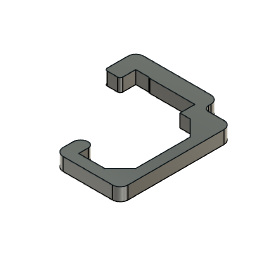
Test frame - motor holders + wheel v4 (Autodesk Fusion 360 archive; units mm, degrees)
design "Single motor Holder"
Autodesk Fusion 360 part; units mm, degrees
note: some values were not read from the file. Chosen so that the rebuilt part matches the saved one: which bodies a step acts on; which face or edge a step refers to. Set by a fixed rule: which sketch regions a step uses.
(part 1 of 2)
sketch "Sketch1" plane through (0, 0, 0) normal (0, 0, 1) x (1, 0, 0)
  line L0 (60.0013, 14) -> (60.0013, 15)
  arc A0 (60.0013, 14) -> (62.0013, 12) centre (62.0013, 14) ccw
  line L1 (51, -27) -> (51, -22.0146)
  line L2 (61, 6) -> (66, 1)
  line L3 (39.0326, 12) -> (39.0326, 11.75)
  line L4 (61, -27) -> (57, -27)
  line L5 (57.0013, 6) -> (61, 6)
  arc A1 (68.0013, -31) -> (71.0013, -28) centre (68.0013, -28) ccw
  line L6 (46, -24.2507) -> (46, -28)
  line L7 (28, 15) -> (28, 6)
  arc A2 (31, 18) -> (28, 15) centre (31, 15) ccw
  line L8 (34, 6) -> (34, 12)
  arc A3 (71.0013, 9) -> (68.0013, 12) centre (68.0013, 9) ccw
  arc A4 (60.0013, 15) -> (57.0013, 18) centre (57.0013, 15) ccw
  arc A5 (46, -28) -> (49, -31) centre (49, -28) ccw
  line L9 (34, 12) -> (39.0326, 12)
  line L10 (68.0013, 12) -> (62.0013, 12)
  line L11 (71.0013, -28) -> (71.0013, 9)
  line L12 (57, 12) -> (57.0013, 12)
  line L13 (39.0326, 11.75) -> (57, 11.75)
  line L14 (49, -31) -> (68.0013, -31)
  line L15 (57.0013, 18) -> (31, 18)
  line L16 (66, 1) -> (66, -22)
  line L17 (28, 6) -> (34, 6)
  line L18 (57, -27) -> (51, -27)
  arc A6 (51, -22.0146) -> (46, -24.2507) centre (49, -24.2507) ccw
  line L19 (66, -22) -> (61, -27)
  line L20 (57.0013, 11.75) -> (57.0013, 6)
  line L21 (57, 11.75) -> (57.0013, 11.75)
  constraint perpendicular L20 L21
extrude "Extrude1" add sketch "Sketch1" along normal blind 5
fillet "Fillet1" radius 1 2 edges at (28, 6, 2.5) (34, 6, 2.5)
fillet "Fillet2" radius 2 1 edges at (51, -22.0146, 2.5)
fillet "Fillet3" radius 1 1 edges at (39.0326, 11.75, 2.5)
sketch "Sketch2" plane through (0, 0, 5) normal (0, 0, 1) x (-1, 0, 0)
  arc A0 (-39.0326, -12) -> (-39.694, -11.75) centre (-39.694, -12.75) ccw
  line L0 (-39.694, -11.75) -> (-57.0013, -11.75)
  line L1 (-57.0013, -11.75) -> (-57.0013, -6)
  line L2 (-57.0013, -6) -> (-61, -6)
  line L3 (-61, -6) -> (-66, -1)
  line L4 (-66, -1) -> (-66, 22)
  line L5 (-66, 22) -> (-61, 27)
  line L6 (-61, 27) -> (-51, 27)
  line L7 (-51, 27) -> (-51, 23.2507)
  arc A1 (-51, 23.2507) -> (-49, 21.2507) centre (-49, 23.2507) ccw
  arc A2 (-49, 21.2507) -> (-46, 24.2507) centre (-49, 24.2507) ccw
  line L8 (-46, 24.2507) -> (-46, 28)
  arc A3 (-46, 28) -> (-49, 31) centre (-49, 28) ccw
  line L9 (-49, 31) -> (-68.0013, 31)
  arc A4 (-68.0013, 31) -> (-71.0013, 28) centre (-68.0013, 28) ccw
  line L10 (-71.0013, 28) -> (-71.0013, -9)
  arc A5 (-71.0013, -9) -> (-68.0013, -12) centre (-68.0013, -9) ccw
  line L11 (-68.0013, -12) -> (-62.0013, -12)
  arc A6 (-60.0013, -14) -> (-62.0013, -12) centre (-62.0013, -14) ccw
  line L12 (-60.0013, -14) -> (-60.0013, -15)
  arc A7 (-60.0013, -15) -> (-57.0013, -18) centre (-57.0013, -15) ccw
  line L13 (-57.0013, -18) -> (-31, -18)
  arc A8 (-31, -18) -> (-28, -15) centre (-31, -15) ccw
  line L14 (-28, -15) -> (-28, -7)
  arc A9 (-28, -7) -> (-29, -6) centre (-29, -7) ccw
  line L15 (-29, -6) -> (-33, -6)
  arc A10 (-33, -6) -> (-34, -7) centre (-33, -7) ccw
  line L16 (-34, -7) -> (-34, -12)
  line L17 (-34, -12) -> (-39.0326, -12)
  line L18 (-66, -1) -> (-67, 0)
  line L19 (-67, 0) -> (-67, 21)
  line L20 (-67, 21) -> (-66, 22)
  constraint coincident L3.end L4.start
  constraint parallel L3 L18
  constraint parallel L4 L19
  constraint coincident L4.end L5.start
  constraint parallel L5 L20
extrude "Extrude2" cut sketch "Sketch2" against normal blind 6 contours L4 L18 L19 L20
sketch "Sketch3" plane through (0, 0, 5) normal (0, 0, 1) x (-1, 0, 0)
  line L0 (-66, -1) -> (-67, 0)
  line L1 (-67, 0) -> (-67, 21)
  line L2 (-67, 21) -> (-61, 27)
  line L3 (-61, 27) -> (-51, 27)
  line L4 (-51, 27) -> (-51, 23.2507)
  arc A0 (-51, 23.2507) -> (-49, 21.2507) centre (-49, 23.2507) ccw
  arc A1 (-49, 21.2507) -> (-46, 24.2507) centre (-49, 24.2507) ccw
  line L5 (-46, 24.2507) -> (-46, 28)
  arc A2 (-46, 28) -> (-49, 31) centre (-49, 28) ccw
  line L6 (-49, 31) -> (-68.0013, 31)
  arc A3 (-68.0013, 31) -> (-71.0013, 28) centre (-68.0013, 28) ccw
  line L7 (-71.0013, 28) -> (-71.0013, -9)
  arc A4 (-71.0013, -9) -> (-68.0013, -12) centre (-68.0013, -9) ccw
  line L8 (-68.0013, -12) -> (-62.0013, -12)
  arc A5 (-60.0013, -14) -> (-62.0013, -12) centre (-62.0013, -14) ccw
  line L9 (-60.0013, -14) -> (-60.0013, -15)
  arc A6 (-60.0013, -15) -> (-57.0013, -18) centre (-57.0013, -15) ccw
  line L10 (-57.0013, -18) -> (-31, -18)
  arc A7 (-31, -18) -> (-28, -15) centre (-31, -15) ccw
  line L11 (-28, -15) -> (-28, -7)
  arc A8 (-28, -7) -> (-29, -6) centre (-29, -7) ccw
  line L12 (-29, -6) -> (-33, -6)
  arc A9 (-33, -6) -> (-34, -7) centre (-33, -7) ccw
  line L13 (-34, -7) -> (-34, -12)
  line L14 (-34, -12) -> (-39.0326, -12)
  arc A10 (-39.0326, -12) -> (-39.694, -11.75) centre (-39.694, -12.75) ccw
  line L15 (-39.694, -11.75) -> (-57.0013, -11.75)
  line L16 (-57.0013, -11.75) -> (-57.0013, -6)
  line L17 (-57.0013, -6) -> (-61, -6)
  line L18 (-61, -6) -> (-66, -1)

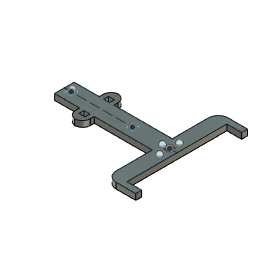
design "Motor Holder"
Autodesk Fusion 360 part; units mm, degrees
sketch "Sketch1" plane through (0, 0, 0) normal (0, 0, 1) x (1, 0, 0)
  line L0 (-40.2212, 51) -> (39.7788, 51)
  line L1 (39.7788, 51) -> (39.7788, -51)
  line L2 (39.7788, -51) -> (-40.2212, -51)
  line L3 (-40.2212, -51) -> (-40.2212, 51)
  line L4 (-40.2212, 51) -> (39.7788, -51) construction
  line L5 (39.7788, 51) -> (-40.2212, -51) construction
  point P0 (-0.2212, 0)
  dimension "d1" = 80
  dimension "d2" = 102
  constraint horizontal L0
  constraint perpendicular L0 L1
  constraint parallel L0 L2
  constraint parallel L1 L3
  constraint coincident L4 P0
  constraint coincident L5 P0
  measures "d1" distance of L1.end L2.end
  measures "d2" distance of L0.end L1.end
extrude "Extrude1" add sketch "Sketch1" along normal blind 6 makes body 1
sketch "Sketch2" plane through (0, 0, 6) normal (0, 0, 1) x (-1, 0, 0)
  line L0 (40.2212, 51) -> (-39.7788, 51)
  line L1 (-39.7788, 51) -> (-39.7788, -51)
  line L2 (-39.7788, -51) -> (40.2212, -51)
  line L3 (40.2212, -51) -> (40.2212, 51)
  line L4 (-39.7788, 0) -> (-39.7788, -10)
  line L5 (-39.7788, -10) -> (20.2212, -10)
  line L6 (20.2212, -10) -> (20.2212, 10)
  line L7 (20.2212, 10) -> (-39.7788, 10)
  line L8 (-25, -10) -> (-25, -45) construction
  line L9 (-24.7788, 10) -> (-24.7788, 45) construction
  line L10 (-24.7788, 10) -> (-24.7788, 45)
  line L11 (-24.7788, 45) -> (-9.7788, 45)
  line L12 (-9.7788, 45) -> (40.2212, 45)
  line L13 (-24.7788, 10) -> (-24.7788, 45)
  line L14 (-25, -10) -> (-25, -45)
  line L15 (40.2212, -45) -> (-25, -45)
  line L16 (-25, -45) -> (-25, -20)
  dimension "d5" = 60
  dimension "d6" = 35
  dimension "d7" = 15
  dimension "d8" = 50
  constraint midpoint L1 L4.start
  constraint coincident L1 L4.end
  constraint parallel L1 L4
  constraint perpendicular L4 L5
  constraint perpendicular L5 L6
  constraint coincident L1 L7.end
  constraint perpendicular L1 L7
  constraint coincident L5 L8.start
  constraint perpendicular L5 L8
  constraint coincident L7 L9.start
  constraint perpendicular L7 L9
  constraint perpendicular L9 L11
  constraint perpendicular L3 L12
  constraint coincident L3 L12.end
  constraint coincident L3 L15.start
  constraint perpendicular L14 L15
  constraint coincident L8 L16.end
  measures "d5" distance of L4.end L5.end
  measures "d6" distance of L8.start L8.end
  measures "d7" distance of L9.end L11.end
  measures "d8" distance of L11.end L12.end
extrude "Extrude2" cut sketch "Sketch2" against normal blind 6 contours L3 L5 L6 L7 L10 L11 L12 L13 L14 L15 L16 bodies 1
sketch "Sketch4" plane through (0, 51, 0) normal (0, 1, 0) x (-1, 0, 0)
  line L0 (-39.7788, 0) -> (40.2212, 0)
  line L1 (40.2212, 0) -> (40.2212, 6)
  line L2 (40.2212, 6) -> (-39.7788, 6)
  line L3 (-39.7788, 6) -> (-39.7788, 0)
  line L4 (-39.7788, 6) -> (-34.7788, 6)
  line L5 (-34.7788, 6) -> (-34.7788, 0)
  line L6 (-34.7788, 0) -> (-39.7788, 0)
  line L7 (-39.7788, 0) -> (-39.7788, 6)
  dimension "d19" = 5
  dimension "d20" = 6
  constraint horizontal L4
  constraint vertical L5
  constraint horizontal L6
  constraint vertical L7
  constraint coincident L2.end L3.start
  measures "d19" distance of L2.end L4.end
  measures "d20" distance of L2.end L0.start
extrude "Extrude4" add sketch "Sketch4" along normal blind 6 contours L0 L2 L3 L4 L5 L6 L7 bodies 1
sketch "Sketch5" plane through (39.7788, 0, 0) normal (1, 0, 0) x (0, 1, 0)
  line L0 (-51, 0) -> (57, 0)
  line L1 (57, 0) -> (57, 6)
  line L2 (57, 6) -> (-51, 6)
  line L3 (-51, 6) -> (-51, 0)
  line L4 (57, 6) -> (51, 6)
  line L5 (51, 6) -> (51, 0)
  line L6 (51, 0) -> (57, 0)
  line L7 (57, 0) -> (57, 6)
  constraint horizontal L4
  constraint vertical L5
  constraint horizontal L6
  constraint vertical L7
  constraint coincident L0 L5.end
  constraint coincident L1.end L2.start
extrude "Extrude5" add sketch "Sketch5" along normal blind 15 contours L0 L1 L2 L4 L5 L6 L7 bodies 1
sketch "Sketch6" plane through (0, 0, 6) normal (0, 0, 1) x (-1, 0, 0)
  line L0 (-24.7788, 45) -> (40.2212, 45)
  line L1 (40.2212, 45) -> (40.2212, 51)
  line L2 (40.2212, 51) -> (-39.7788, 51)
  line L3 (-39.7788, 51) -> (-39.7788, -51)
  line L4 (-39.7788, -51) -> (-54.7788, -51)
  line L5 (-54.7788, -51) -> (-54.7788, -57)
  line L6 (-54.7788, -57) -> (-34.7788, -57)
  line L7 (-34.7788, -57) -> (-34.7788, -51)
  line L8 (-34.7788, -51) -> (40.2212, -51)
  line L9 (40.2212, -51) -> (40.2212, -45)
  line L10 (40.2212, -45) -> (-25, -45)
  line L11 (-25, -45) -> (-25, -10)
  line L12 (-25, -10) -> (20.2212, -10)
  line L13 (20.2212, -10) -> (20.2212, 10)
  line L14 (20.2212, 10) -> (-24.7788, 10)
  line L15 (-24.7788, 10) -> (-24.7788, 45)
  line L16 (-34.7788, -57) -> (-28.7788, -51)
  line L17 (-34.7788, -57) -> (-26.2935, -57) construction
  dimension "d25" = 45
  constraint horizontal L17
  constraint coincident L6.end L7.start
  constraint coincident L8 L16.end
  measures "d25" angle of L16 L17
extrude "Extrude6" add sketch "Sketch6" against normal blind 6 contours L7 L8 L16 bodies 1
sketch "Sketch7" plane through (0, -51, 0) normal (0, -1, 0) x (1, 0, 0)
  line L0 (-40.2212, 0) -> (39.7788, 0)
  line L1 (39.7788, 0) -> (39.7788, 6)
  line L2 (39.7788, 6) -> (-40.2212, 6)
  line L3 (-40.2212, 6) -> (-40.2212, 0)
  line L4 (39.7788, 6) -> (34.7788, 6) construction
  line L5 (34.7788, 6) -> (34.7788, 0) construction
  line L6 (34.7788, 0) -> (39.7788, 0) construction
  line L7 (39.7788, 0) -> (39.7788, 6) construction
  line L8 (34.7788, 6) -> (39.7788, 6)
  line L9 (39.7788, 6) -> (39.7788, 0)
  line L10 (39.7788, 0) -> (34.7788, 0)
  line L11 (34.7788, 0) -> (34.7788, 6)
  dimension "d28" = 5
  constraint horizontal L4
  constraint vertical L5
  constraint horizontal L6
  constraint vertical L7
  constraint coincident L0 L5.end
  constraint coincident L1.end L2.start
  constraint horizontal L8
  constraint vertical L9
  constraint horizontal L10
  constraint vertical L11
  constraint coincident L0.end L1.start
  measures "d28" distance of L1.end L4.end
extrude "Extrude7" add sketch "Sketch7" along normal blind 6 contours L0 L1 L2 L8 L9 L10 L11 bodies 1
sketch "Sketch8" plane through (39.7788, 0, 0) normal (1, 0, 0) x (0, 1, 0)
  line L0 (51, 0) -> (51, 6)
  line L1 (51, 6) -> (-57, 6)
  line L2 (-57, 6) -> (-57, 0)
  line L3 (-57, 0) -> (51, 0)
  line L4 (-57, 6) -> (-51, 6)
  line L5 (-51, 6) -> (-51, 0)
  line L6 (-51, 0) -> (-57, 0)
  line L7 (-57, 0) -> (-57, 6)
  constraint horizontal L4
  constraint vertical L5
  constraint horizontal L6
  constraint vertical L7
  constraint coincident L3 L5.end
  constraint coincident L1.end L2.start
extrude "Extrude8" add sketch "Sketch8" along normal blind 15 contours L1 L2 L3 L4 L5 L6 L7 bodies 1
sketch "Sketch9" plane through (0, 0, 6) normal (0, 0, 1) x (-1, 0, 0)
  line L0 (-24.7788, 45) -> (40.2212, 45)
  line L1 (40.2212, 45) -> (40.2212, 51)
  line L2 (40.2212, 51) -> (-34.7788, 51)
  line L3 (-34.7788, 51) -> (-34.7788, 57)
  line L4 (-34.7788, 57) -> (-54.7788, 57)
  line L5 (-54.7788, 57) -> (-54.7788, 51)
  line L6 (-54.7788, 51) -> (-39.7788, 51)
  line L7 (-39.7788, 51) -> (-39.7788, -51)
  line L8 (-39.7788, -51) -> (-54.7788, -51)
  line L9 (-54.7788, -51) -> (-54.7788, -57)
  line L10 (-54.7788, -57) -> (-34.7788, -57)
  line L11 (-34.7788, -57) -> (-28.7788, -51)
  line L12 (-28.7788, -51) -> (40.2212, -51)
  line L13 (40.2212, -51) -> (40.2212, -45)
  line L14 (40.2212, -45) -> (-25, -45)
  line L15 (-25, -45) -> (-25, -10)
  line L16 (-25, -10) -> (20.2212, -10)
  line L17 (20.2212, -10) -> (20.2212, 10)
  line L18 (20.2212, 10) -> (-24.7788, 10)
  line L19 (-24.7788, 10) -> (-24.7788, 45)
  line L20 (-34.7788, 57) -> (-28.7788, 51)
  line L21 (-34.7788, 57) -> (-26.2935, 57) construction
  dimension "d33" = 45
  constraint horizontal L21
  constraint coincident L3.end L4.start
  constraint coincident L2 L20.end
  measures "d33" angle of L20 L21
extrude "Extrude9" add sketch "Sketch9" against normal blind 6 contours L2 L3 L20 bodies 1
sketch "Sketch10" plane through (0, 0, 6) normal (0, 0, 1) x (-1, 0, 0)
  line L0 (-24.7788, 45) -> (40.2212, 45)
  line L1 (40.2212, 45) -> (40.2212, 51)
  line L2 (40.2212, 51) -> (-28.7788, 51)
  line L3 (-28.7788, 51) -> (-34.7788, 57)
  line L4 (-34.7788, 57) -> (-54.7788, 57)
  line L5 (-54.7788, 57) -> (-54.7788, 51)
  line L6 (-54.7788, 51) -> (-39.7788, 51)
  line L7 (-39.7788, 51) -> (-39.7788, -51)
  line L8 (-39.7788, -51) -> (-54.7788, -51)
  line L9 (-54.7788, -51) -> (-54.7788, -57)
  line L10 (-54.7788, -57) -> (-34.7788, -57)
  line L11 (-34.7788, -57) -> (-28.7788, -51)
  line L12 (-28.7788, -51) -> (40.2212, -51)
  line L13 (40.2212, -51) -> (40.2212, -45)
  line L14 (40.2212, -45) -> (-25, -45)
  line L15 (-25, -45) -> (-25, -10)
  line L16 (-25, -10) -> (20.2212, -10)
  line L17 (20.2212, -10) -> (20.2212, 10)
  line L18 (20.2212, 10) -> (-24.7788, 10)
  line L19 (-24.7788, 10) -> (-24.7788, 45)
  line L20 (-25, -10) -> (35, -10) construction
  line L21 (35, -10) -> (35, 10) construction
  line L22 (35, 10) -> (20.2212, 10) construction
  line L23 (35, -10) -> (20.2212, -10) construction
  line L24 (20.2212, -10) -> (20.2212, 10) construction
  line L25 (20.2212, 10) -> (35, 10) construction
  line L26 (35, 10) -> (35, -10) construction
  line L27 (35, 10) -> (20.2212, 10)
  line L28 (20.2212, 10) -> (20.2212, -10)
  line L29 (20.2212, -10) -> (35, -10)
  line L30 (35, -10) -> (35, 10)
  constraint coincident L15.end L16.start
  constraint perpendicular L17 L20
  constraint perpendicular L20 L21
  constraint coincident L17.end L18.start
  constraint perpendicular L17 L22
  constraint horizontal L23
  constraint vertical L24
  constraint horizontal L25
  constraint vertical L26
  constraint horizontal L27
  constraint vertical L28
  constraint horizontal L29
  constraint vertical L30
  constraint coincident L16.end L17.start
extrude "Extrude10" add sketch "Sketch10" against normal blind 6 separate body contours L17 L27 L28 L29 L30 makes body 2
sketch "Sketch12" plane through (-35, 0, 0) normal (-1, 0, 0) x (0, -1, 0)
  line L0 (10, 6) -> (-10, 6)
  line L1 (-10, 6) -> (-10, 0)
  line L2 (-10, 0) -> (10, 0)
  line L3 (10, 0) -> (10, 6)
extrude "Extrude11" add sketch "Sketch12" along normal blind 40 bodies 2
combine "Combine1" operation add target body 2 tool bodies 1
sketch "Sketch13" plane through (0, 0, 6) normal (0, 0, 1) x (-1, 0, 0)
  line L0 (75, 10) -> (-24.7788, 10)
  line L1 (-24.7788, 10) -> (-24.7788, 45)
  line L2 (-24.7788, 45) -> (40.2212, 45)
  line L3 (40.2212, 45) -> (40.2212, 51)
  line L4 (40.2212, 51) -> (-28.7788, 51)
  line L5 (-28.7788, 51) -> (-34.7788, 57)
  line L6 (-34.7788, 57) -> (-54.7788, 57)
  line L7 (-54.7788, 57) -> (-54.7788, 51)
  line L8 (-54.7788, 51) -> (-39.7788, 51)
  line L9 (-39.7788, 51) -> (-39.7788, -51)
  line L10 (-39.7788, -51) -> (-54.7788, -51)
  line L11 (-54.7788, -51) -> (-54.7788, -57)
  line L12 (-54.7788, -57) -> (-34.7788, -57)
  line L13 (-34.7788, -57) -> (-28.7788, -51)
  line L14 (-28.7788, -51) -> (40.2212, -51)
  line L15 (40.2212, -51) -> (40.2212, -45)
  line L16 (40.2212, -45) -> (-25, -45)
  line L17 (-25, -45) -> (-25, -10)
  line L18 (-25, -10) -> (75, -10)
  line L19 (75, -10) -> (75, 10)
  line L20 (-28.7788, 51) -> (-24.7788, 45)
  line L21 (-28.7788, -51) -> (-25, -45)
  constraint coincident L4.end L5.start
  constraint coincident L1.end L2.start
  constraint coincident L13.end L14.start
  constraint coincident L16.end L17.start
extrude "Extrude12" cut sketch "Sketch13" against normal blind 11 contours L2 L3 L4 L20 | L14 L15 L16 L21 bodies 2
sketch "Sketch14" plane through (0, 0, 6) normal (0, 0, 1) x (-1, 0, 0)
  line L0 (-24.7788, 45) -> (-28.7788, 51)
  line L1 (-28.7788, 51) -> (-34.7788, 57)
  line L2 (-34.7788, 57) -> (-54.7788, 57)
  line L3 (-54.7788, 57) -> (-54.7788, 51)
  line L4 (-54.7788, 51) -> (-39.7788, 51)
  line L5 (-39.7788, 51) -> (-39.7788, -51)
  line L6 (-39.7788, -51) -> (-54.7788, -51)
  line L7 (-54.7788, -51) -> (-54.7788, -57)
  line L8 (-54.7788, -57) -> (-34.7788, -57)
  line L9 (-34.7788, -57) -> (-28.7788, -51)
  line L10 (-28.7788, -51) -> (-25, -45)
  line L11 (-25, -45) -> (-25, -10)
  line L12 (-25, -10) -> (75, -10)
  line L13 (75, -10) -> (75, 10)
  line L14 (75, 10) -> (-24.7788, 10)
  line L15 (-24.7788, 10) -> (-24.7788, 45)
  line L16 (-25, -45) -> (-25, -57)
  line L17 (-25, -57) -> (-34.7788, -57)
  line L18 (-24.7788, 45) -> (-24.7788, 57)
  line L19 (-24.7788, 57) -> (-34.7788, 57)
  constraint coincident L10.end L11.start
  constraint parallel L11 L16
  constraint coincident L8.end L9.start
  constraint perpendicular L16 L17
  constraint coincident L0.start L15.end
  constraint perpendicular L2 L18
  constraint coincident L1.end L2.start
  constraint perpendicular L18 L19
extrude "Extrude13" add sketch "Sketch14" against normal blind 6 contours L0 L1 L18 L19 | L9 L10 L16 L17 bodies 2
fillet "Fillet1" radius 10 2 edges at (24.7788, -57, 3) (25, 57, 3) on bodies 2
sketch "Sketch15" plane through (0, 0, 6) normal (0, 0, 1) x (-1, 0, 0)
  arc A0 (-35, -57) -> (-25, -47) centre (-35, -47) ccw
  line L0 (-25, -47) -> (-25, -10)
  line L1 (-25, -10) -> (75, -10)
  line L2 (75, -10) -> (75, 10)
  line L3 (75, 10) -> (-24.7788, 10)
  line L4 (-24.7788, 10) -> (-24.7788, 47)
  arc A1 (-24.7788, 47) -> (-34.7788, 57) centre (-34.7788, 47) ccw
  line L5 (-34.7788, 57) -> (-54.7788, 57)
  line L6 (-54.7788, 57) -> (-54.7788, 51)
  line L7 (-54.7788, 51) -> (-39.7788, 51)
  line L8 (-39.7788, 51) -> (-39.7788, -51)
  line L9 (-39.7788, -51) -> (-54.7788, -51)
  line L10 (-54.7788, -51) -> (-54.7788, -57)
  line L11 (-54.7788, -57) -> (-35, -57)
  line L12 (-39.7788, 0) -> (-25, 0) construction
  line L13 (-32.3894, 10.2212) -> (-32.3894, -10) construction
  line L14 (-29.8894, 3) -> (-34.8894, 3)
  line L15 (-34.8894, 3) -> (-34.8894, -3)
  line L16 (-34.8894, -3) -> (-29.8894, -3)
  line L17 (-29.8894, -3) -> (-29.8894, 3)
  line L18 (-29.8894, 3) -> (-34.8894, -3) construction
  line L19 (-34.8894, 3) -> (-29.8894, -3) construction
  line L20 (75, 0) -> (8, 0) construction
  line L21 (8, 0) -> (5.5, 0) construction
  line L22 (8, -3) -> (3, -3)
  line L23 (3, -3) -> (3, 3)
  line L24 (3, 3) -> (8, 3)
  line L25 (8, 3) -> (8, -3)
  line L26 (8, -3) -> (3, 3) construction
  line L27 (3, -3) -> (8, 3) construction
  line L28 (75, 0) -> (70, 0) construction
  line L29 (70, 0) -> (70, -3) construction
  line L30 (70.5, -3) -> (65.5, -3)
  line L31 (65.5, -3) -> (65.5, 3)
  line L32 (65.5, 3) -> (70.5, 3)
  line L33 (70.5, 3) -> (70.5, -3)
  line L34 (70.5, -3) -> (65.5, 3) construction
  line L35 (65.5, -3) -> (70.5, 3) construction
  point P0 (-32.3894, 0)
  point P1 (5.5, 0)
  point P2 (68, 0)
  dimension "d53" = 5
  dimension "d54" = 6
  dimension "d59" = 2.5
  dimension "d62" = 5
  constraint midpoint L8 L12.start
  constraint perpendicular L8 L12
  constraint perpendicular L12 L13
  constraint horizontal L14
  constraint perpendicular L14 L15
  constraint parallel L14 L16
  constraint parallel L15 L17
  constraint coincident L18 P0
  constraint coincident L19 P0
  constraint midpoint L12 P0
  constraint midpoint L2 L20.start
  constraint parallel L20 L21
  constraint horizontal L22
  constraint perpendicular L22 L23
  constraint parallel L22 L24
  constraint parallel L23 L25
  constraint coincident L26 P1
  constraint coincident L27 P1
  constraint coincident P1 L21.end
  constraint coincident L20 L28.end
  constraint perpendicular L2 L28
  constraint perpendicular L28 L29
  constraint horizontal L30
  constraint perpendicular L30 L31
  constraint parallel L30 L32
  constraint parallel L31 L33
  constraint coincident L34 P2
  constraint coincident L35 P2
  constraint coincident L20 P2
  measures "d53" distance of L15.end L16.end
  measures "d54" distance of L14.end L15.end
  measures "d59" distance of L20.end P1
  measures "d62" distance of L31.end L32.end
extrude "Extrude15" cut sketch "Sketch15" against normal blind 8 contours L14 L15 L16 L17 bodies 2
extrude "Extrude16" cut sketch "Sketch15" against normal blind 6 contours L14 L15 L16 L17 | L22 L23 L24 L25 bodies 2
extrude "Extrude17" cut sketch "Sketch15" against normal blind 6 contours L30 L31 L32 L33 bodies 2
sketch "Sketch16" plane through (0, -10, 0) normal (0, -1, 0) x (1, 0, 0)
  line L0 (24.7788, 6) -> (-75, 6)
  line L1 (-75, 6) -> (-75, 0)
  line L2 (-75, 0) -> (24.7788, 0)
  line L3 (24.7788, 0) -> (24.7788, 6)
  line L4 (-75, 3) -> (-42, 3) construction
  line L5 (-42, 3) -> (-9, 3) construction
  line L6 (-44.5, 6) -> (-39.5, 6) construction
  line L7 (-39.5, 6) -> (-39.5, 0) construction
  line L8 (-39.5, 0) -> (-44.5, 0) construction
  line L9 (-44.5, 0) -> (-44.5, 6) construction
  line L10 (-44.5, 6) -> (-39.5, 0) construction
  line L11 (-39.5, 6) -> (-44.5, 0) construction
  line L12 (-44.5, 6) -> (-49.5, 6)
  line L13 (-49.5, 6) -> (-49.5, 0)
  line L14 (-49.5, 0) -> (-44.5, 0)
  line L15 (-44.5, 0) -> (-44.5, 6)
  line L16 (-39.5, 6) -> (-34.5, 6)
  line L17 (-34.5, 6) -> (-34.5, 0)
  line L18 (-34.5, 0) -> (-39.5, 0)
  line L19 (-39.5, 0) -> (-39.5, 6)
  point P0 (-42, 3)
  dimension "d65" = 33
  dimension "d66" = 33
  dimension "d67" = 5
  dimension "d68" = 5
  dimension "d69" = 6
  dimension "d70" = 5
  dimension "d71" = 6
  constraint midpoint L1 L4.start
  constraint perpendicular L1 L4
  constraint perpendicular L1 L5
  constraint horizontal L6
  constraint perpendicular L6 L7
  constraint parallel L6 L8
  constraint parallel L7 L9
  constraint coincident L10 P0
  constraint coincident L11 P0
  constraint coincident P0 L4.end
  constraint horizontal L12
  constraint vertical L13
  constraint horizontal L14
  constraint vertical L15
  constraint horizontal L16
  constraint vertical L17
  constraint horizontal L18
  constraint vertical L19
  measures "d65" distance of L4.start P0
  measures "d66" distance of P0 L5.end
  measures "d67" distance of L7.end L8.end
  measures "d68" distance of L6.start L12.end
  measures "d69" distance of L6.start L8.end
  measures "d70" distance of L6.end L16.end
  measures "d71" distance of L6.end L7.end
extrude "Extrude18" add sketch "Sketch16" along normal blind 12 contours L0 L2 L16 L17 L18 L19 | L0 L2 L12 L13 L14 L15 bodies 2
sketch "Sketch17" plane through (-39.5, 0, 0) normal (-1, 0, 0) x (0, -1, 0)
  line L0 (10, 6) -> (10, 0)
  line L1 (10, 0) -> (22, 0)
  line L2 (22, 0) -> (22, 6)
  line L3 (22, 6) -> (10, 6)
  line L4 (22, 6) -> (16, 6)
  line L5 (16, 6) -> (16, 0)
  line L6 (16, 0) -> (22, 0)
  line L7 (22, 0) -> (22, 6)
  dimension "d74" = 6
  constraint horizontal L4
  constraint vertical L5
  constraint horizontal L6
  constraint vertical L7
  constraint coincident L2.end L3.start
  measures "d74" distance of L2.end L4.end
extrude "Extrude19" add sketch "Sketch17" along normal blind 5 contours L1 L2 L3 L4 L5 L6 L7 bodies 2
mirror "Mirror1" about plane through (0, 0, 0) normal (0, 1, 0) of "Extrude18", "Extrude19"
sketch "Sketch18" plane through (0, 0, 6) normal (0, 0, 1) x (-1, 0, 0)
  line L0 (39.5, -16) -> (39.5, -10)
  line L1 (39.5, -10) -> (44.5, -10)
  line L2 (44.5, -10) -> (44.5, -16)
  line L3 (44.5, -16) -> (39.5, -16)
  line L4 (34.5, -22) -> (49.5, -22)
  line L5 (49.5, -22) -> (49.5, -10)
  line L6 (49.5, -10) -> (75, -10)
  line L7 (75, -10) -> (75, 10)
  line L8 (75, 10) -> (49.5, 10)
  line L9 (49.5, 10) -> (49.5, 22)
  line L10 (49.5, 22) -> (34.5, 22)
  line L11 (34.5, 22) -> (34.5, 10)
  line L12 (34.5, 10) -> (-24.7788, 10)
  line L13 (-24.7788, 10) -> (-24.7788, 47)
  arc A0 (-24.7788, 47) -> (-34.7788, 57) centre (-34.7788, 47) ccw
  line L14 (-34.7788, 57) -> (-54.7788, 57)
  line L15 (-54.7788, 57) -> (-54.7788, 51)
  line L16 (-54.7788, 51) -> (-39.7788, 51)
  line L17 (-39.7788, 51) -> (-39.7788, -51)
  line L18 (-39.7788, -51) -> (-54.7788, -51)
  line L19 (-54.7788, -51) -> (-54.7788, -57)
  line L20 (-54.7788, -57) -> (-35, -57)
  arc A1 (-35, -57) -> (-25, -47) centre (-35, -47) ccw
  line L21 (-25, -47) -> (-25, -10)
  line L22 (-25, -10) -> (34.5, -10)
  line L23 (34.5, -10) -> (34.5, -22)
  line L24 (65.5, -3) -> (65.5, 3)
  line L25 (65.5, 3) -> (70.5, 3)
  line L26 (70.5, 3) -> (70.5, -3)
  line L27 (70.5, -3) -> (65.5, -3)
  line L28 (3, -3) -> (3, 3)
  line L29 (3, 3) -> (8, 3)
  line L30 (8, 3) -> (8, -3)
  line L31 (8, -3) -> (3, -3)
  line L32 (-34.8894, 3) -> (-29.8894, 3)
  line L33 (-29.8894, 3) -> (-29.8894, -3)
  line L34 (-29.8894, -3) -> (-34.8894, -3)
  line L35 (-34.8894, -3) -> (-34.8894, 3)
  line L36 (39.5, 16) -> (44.5, 16)
  line L37 (44.5, 16) -> (44.5, 10)
  line L38 (44.5, 10) -> (39.5, 10)
  line L39 (39.5, 10) -> (39.5, 16)
  line L40 (45, 10) -> (39, 10)
  line L41 (39, 10) -> (39, 15)
  line L42 (39, 15) -> (45, 15)
  line L43 (45, 15) -> (45, 10)
  line L44 (44.5, 15) -> (39.5, 15)
  line L45 (39.5, 15) -> (39.5, 16)
  line L46 (39.5, 16) -> (44.5, 16)
  line L47 (44.5, 16) -> (44.5, 15)
  dimension "d79" = 6
  dimension "d80" = 5
  constraint horizontal L40
  constraint vertical L41
  constraint horizontal L42
  constraint vertical L43
  constraint horizontal L44
  constraint vertical L45
  constraint horizontal L46
  constraint vertical L47
  constraint coincident L36.start L39.end
  constraint coincident L42 L44.start
  constraint coincident L37 L44.start
  measures "d79" distance of L40.start L40.end
  measures "d80" distance of L40.start L42.end
extrude "Extrude20" cut sketch "Sketch18" against normal blind 7 contours L39 L40 L41 L42 | L37 L40 L42 L43 bodies 2
sketch "Sketch19" plane through (0, 0, 6) normal (0, 0, 1) x (-1, 0, 0)
  line L0 (45, 10) -> (39, 10)
  line L1 (39, 10) -> (39, 15)
  line L2 (39, 15) -> (39.5, 15)
  line L3 (39.5, 15) -> (39.5, 16)
  line L4 (39.5, 16) -> (44.5, 16)
  line L5 (44.5, 16) -> (44.5, 15)
  line L6 (44.5, 15) -> (45, 15)
  line L7 (45, 15) -> (45, 10)
  line L8 (39.5, -16) -> (39.5, -10)
  line L9 (39.5, -10) -> (44.5, -10)
  line L10 (44.5, -10) -> (44.5, -16)
  line L11 (44.5, -16) -> (39.5, -16)
  line L12 (34.5, -22) -> (49.5, -22)
  line L13 (49.5, -22) -> (49.5, -10)
  line L14 (49.5, -10) -> (75, -10)
  line L15 (75, -10) -> (75, 10)
  line L16 (75, 10) -> (49.5, 10)
  line L17 (49.5, 10) -> (49.5, 22)
  line L18 (49.5, 22) -> (34.5, 22)
  line L19 (34.5, 22) -> (34.5, 10)
  line L20 (34.5, 10) -> (-24.7788, 10)
  line L21 (-24.7788, 10) -> (-24.7788, 47)
  arc A0 (-24.7788, 47) -> (-34.7788, 57) centre (-34.7788, 47) ccw
  line L22 (-34.7788, 57) -> (-54.7788, 57)
  line L23 (-54.7788, 57) -> (-54.7788, 51)
  line L24 (-54.7788, 51) -> (-39.7788, 51)
  line L25 (-39.7788, 51) -> (-39.7788, -51)
  line L26 (-39.7788, -51) -> (-54.7788, -51)
  line L27 (-54.7788, -51) -> (-54.7788, -57)
  line L28 (-54.7788, -57) -> (-35, -57)
  arc A1 (-35, -57) -> (-25, -47) centre (-35, -47) ccw
  line L29 (-25, -47) -> (-25, -10)
  line L30 (-25, -10) -> (34.5, -10)
  line L31 (34.5, -10) -> (34.5, -22)
  line L32 (65.5, -3) -> (65.5, 3)
  line L33 (65.5, 3) -> (70.5, 3)
  line L34 (70.5, 3) -> (70.5, -3)
  line L35 (70.5, -3) -> (65.5, -3)
  line L36 (3, -3) -> (3, 3)
  line L37 (3, 3) -> (8, 3)
  line L38 (8, 3) -> (8, -3)
  line L39 (8, -3) -> (3, -3)
  line L40 (-34.8894, 3) -> (-29.8894, 3)
  line L41 (-29.8894, 3) -> (-29.8894, -3)
  line L42 (-29.8894, -3) -> (-34.8894, -3)
  line L43 (-34.8894, -3) -> (-34.8894, 3)
  line L44 (44.5, 15) -> (39.5, 15)
  line L45 (39.5, 15) -> (39.5, 16)
  line L46 (39.5, 16) -> (44.5, 16)
  line L47 (44.5, 16) -> (44.5, 15)
  constraint horizontal L44
  constraint vertical L45
  constraint horizontal L46
  constraint vertical L47
  constraint coincident L3.end L4.start
  constraint coincident L5.end L6.start
extrude "Extrude21" add sketch "Sketch19" against normal blind 6 contours L3 L4 L5 L44 L45 L46 L47 bodies 2
sketch "Sketch20" plane through (0, 0, 6) normal (0, 0, 1) x (-1, 0, 0)
  line L0 (45, 10) -> (39, 10)
  line L1 (39, 10) -> (39, 15)
  line L2 (39, 15) -> (45, 15)
  line L3 (45, 15) -> (45, 10)
  line L4 (39.5, -16) -> (39.5, -10)
  line L5 (39.5, -10) -> (44.5, -10)
  line L6 (44.5, -10) -> (44.5, -16)
  line L7 (44.5, -16) -> (39.5, -16)
  line L8 (34.5, -22) -> (49.5, -22)
  line L9 (49.5, -22) -> (49.5, -10)
  line L10 (49.5, -10) -> (75, -10)
  line L11 (75, -10) -> (75, 10)
  line L12 (75, 10) -> (49.5, 10)
  line L13 (49.5, 10) -> (49.5, 22)
  line L14 (49.5, 22) -> (34.5, 22)
  line L15 (34.5, 22) -> (34.5, 10)
  line L16 (34.5, 10) -> (-24.7788, 10)
  line L17 (-24.7788, 10) -> (-24.7788, 47)
  arc A0 (-24.7788, 47) -> (-34.7788, 57) centre (-34.7788, 47) ccw
  line L18 (-34.7788, 57) -> (-54.7788, 57)
  line L19 (-54.7788, 57) -> (-54.7788, 51)
  line L20 (-54.7788, 51) -> (-39.7788, 51)
  line L21 (-39.7788, 51) -> (-39.7788, -51)
  line L22 (-39.7788, -51) -> (-54.7788, -51)
  line L23 (-54.7788, -51) -> (-54.7788, -57)
  line L24 (-54.7788, -57) -> (-35, -57)
  arc A1 (-35, -57) -> (-25, -47) centre (-35, -47) ccw
  line L25 (-25, -47) -> (-25, -10)
  line L26 (-25, -10) -> (34.5, -10)
  line L27 (34.5, -10) -> (34.5, -22)
  line L28 (65.5, -3) -> (65.5, 3)
  line L29 (65.5, 3) -> (70.5, 3)
  line L30 (70.5, 3) -> (70.5, -3)
  line L31 (70.5, -3) -> (65.5, -3)
  line L32 (3, -3) -> (3, 3)
  line L33 (3, 3) -> (8, 3)
  line L34 (8, 3) -> (8, -3)
  line L35 (8, -3) -> (3, -3)
  line L36 (-34.8894, 3) -> (-29.8894, 3)
  line L37 (-29.8894, 3) -> (-29.8894, -3)
  line L38 (-29.8894, -3) -> (-34.8894, -3)
  line L39 (-34.8894, -3) -> (-34.8894, 3)
  line L40 (39, -10) -> (45, -10)
  line L41 (45, -10) -> (45, -15)
  line L42 (45, -15) -> (39, -15)
  line L43 (39, -15) -> (39, -10)
  dimension "d85" = 5
  constraint horizontal L40
  constraint vertical L41
  constraint horizontal L42
  constraint vertical L43
  measures "d85" distance of L40.start L42.end
extrude "Extrude22" cut sketch "Sketch20" against normal blind 6 contours L4 L40 L42 L43 | L6 L40 L41 L42 bodies 2
sketch "Sketch21" plane through (0, 0, 6) normal (0, 0, 1) x (-1, 0, 0)
  line L0 (-34.8894, 3) -> (-29.8894, 3)
  line L1 (-29.8894, 3) -> (-29.8894, -3)
  line L2 (-29.8894, -3) -> (-34.8894, -3)
  line L3 (-34.8894, -3) -> (-34.8894, 3)
  line L4 (3, -3) -> (3, 3)
  line L5 (3, 3) -> (8, 3)
  line L6 (8, 3) -> (8, -3)
  line L7 (8, -3) -> (3, -3)
  line L8 (65.5, -3) -> (65.5, 3)
  line L9 (65.5, 3) -> (70.5, 3)
  line L10 (70.5, 3) -> (70.5, -3)
  line L11 (70.5, -3) -> (65.5, -3)
  line L12 (34.5, -22) -> (49.5, -22)
  line L13 (49.5, -22) -> (49.5, -10)
  line L14 (49.5, -10) -> (75, -10)
  line L15 (75, -10) -> (75, 10)
  line L16 (75, 10) -> (49.5, 10)
  line L17 (49.5, 10) -> (49.5, 22)
  line L18 (49.5, 22) -> (34.5, 22)
  line L19 (34.5, 22) -> (34.5, 10)
  line L20 (34.5, 10) -> (-24.7788, 10)
  line L21 (-24.7788, 10) -> (-24.7788, 47)
  arc A0 (-24.7788, 47) -> (-34.7788, 57) centre (-34.7788, 47) ccw
  line L22 (-34.7788, 57) -> (-54.7788, 57)
  line L23 (-54.7788, 57) -> (-54.7788, 51)
  line L24 (-54.7788, 51) -> (-39.7788, 51)
  line L25 (-39.7788, 51) -> (-39.7788, -51)
  line L26 (-39.7788, -51) -> (-54.7788, -51)
  line L27 (-54.7788, -51) -> (-54.7788, -57)
  line L28 (-54.7788, -57) -> (-35, -57)
  arc A1 (-35, -57) -> (-25, -47) centre (-35, -47) ccw
  line L29 (-25, -47) -> (-25, -10)
  line L30 (-25, -10) -> (34.5, -10)
  line L31 (34.5, -10) -> (34.5, -22)
  line L32 (39.5, -15) -> (39, -15)
  line L33 (39, -15) -> (39, -10)
  line L34 (39, -10) -> (45, -10)
  line L35 (45, -10) -> (45, -15)
  line L36 (45, -15) -> (44.5, -15)
  line L37 (44.5, -15) -> (44.5, -16)
  line L38 (44.5, -16) -> (39.5, -16)
  line L39 (39.5, -16) -> (39.5, -15)
  line L40 (45, 10) -> (39, 10)
  line L41 (39, 10) -> (39, 15)
  line L42 (39, 15) -> (45, 15)
  line L43 (45, 15) -> (45, 10)
  line L44 (39.5, -15) -> (44.5, -15)
  line L45 (44.5, -15) -> (44.5, -16)
  line L46 (44.5, -16) -> (39.5, -16)
  line L47 (39.5, -16) -> (39.5, -15)
  constraint horizontal L44
  constraint vertical L45
  constraint horizontal L46
  constraint vertical L47
  constraint coincident L37.end L38.start
  constraint coincident L32.start L39.end
extrude "Extrude23" add sketch "Sketch21" against normal blind 6 contours L37 L38 L39 L44 L45 L46 L47 bodies 2
fillet "Fillet2" radius 8 8 edges at (-42, -22, 6) (-42, 22, 6) (-42, 22, 0) (-42, -22, 0) (-49.5, 22, 3) (-34.5, 22, 3) (-49.5, -22, 3) (-34.5, -22, 3) on bodies 2
sketch "Sketch22" plane through (0, 0, 6) normal (0, 0, 1) x (-1, 0, 0)
  arc A0 (49.5, 14.0627) -> (42.5, 22) centre (41.5, 14.0627) ccw
  arc A1 (42.5, 22) -> (34.5, 14) centre (42.5, 14) ccw
  line L0 (34.5, 14) -> (34.5, 10)
  line L1 (34.5, 10) -> (-24.7788, 10)
  line L2 (-24.7788, 10) -> (-24.7788, 47)
  arc A2 (-24.7788, 47) -> (-34.7788, 57) centre (-34.7788, 47) ccw
  line L3 (-34.7788, 57) -> (-54.7788, 57)
  line L4 (-54.7788, 57) -> (-54.7788, 51)
  line L5 (-54.7788, 51) -> (-39.7788, 51)
  line L6 (-39.7788, 51) -> (-39.7788, -51)
  line L7 (-39.7788, -51) -> (-54.7788, -51)
  line L8 (-54.7788, -51) -> (-54.7788, -57)
  line L9 (-54.7788, -57) -> (-35, -57)
  arc A3 (-35, -57) -> (-25, -47) centre (-35, -47) ccw
  line L10 (-25, -47) -> (-25, -10)
  line L11 (-25, -10) -> (34.5, -10)
  line L12 (34.5, -10) -> (34.5, -14)
  arc A4 (34.5, -14) -> (42.5, -22) centre (42.5, -14) ccw
  arc A5 (42.5, -22) -> (49.5, -14.0627) centre (41.5, -14.0627) ccw
  line L13 (49.5, -14.0627) -> (49.5, -10)
  line L14 (49.5, -10) -> (75, -10)
  line L15 (75, -10) -> (75, 10)
  line L16 (75, 10) -> (49.5, 10)
  line L17 (49.5, 10) -> (49.5, 14.0627)
  line L18 (-34.8894, 3) -> (-29.8894, 3)
  line L19 (-29.8894, 3) -> (-29.8894, -3)
  line L20 (-29.8894, -3) -> (-34.8894, -3)
  line L21 (-34.8894, -3) -> (-34.8894, 3)
  line L22 (3, -3) -> (3, 3)
  line L23 (3, 3) -> (8, 3)
  line L24 (8, 3) -> (8, -3)
  line L25 (8, -3) -> (3, -3)
  line L26 (65.5, -3) -> (65.5, 3)
  line L27 (65.5, 3) -> (70.5, 3)
  line L28 (70.5, 3) -> (70.5, -3)
  line L29 (70.5, -3) -> (65.5, -3)
  line L30 (45, -15) -> (39, -15)
  line L31 (39, -15) -> (39, -10)
  line L32 (39, -10) -> (45, -10)
  line L33 (45, -10) -> (45, -15)
  line L34 (45, 10) -> (39, 10)
  line L35 (39, 10) -> (39, 15)
  line L36 (39, 15) -> (45, 15)
  line L37 (45, 15) -> (45, 10)

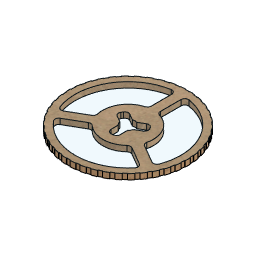
design "wheel + hub hole"
Autodesk Fusion 360 part; units mm, degrees
sketch "Sketch1" plane through (0, 0, 0) normal (0, 0, 1) x (1, 0, 0)
  line L0 (-14.6554, 9.616) -> (-15.6554, 7.884)
  arc A0 (14.6554, 9.616) -> (9.1913, 11.0801) centre (11.1913, 7.616) ccw
  line L1 (-1, -17.5) -> (1, -17.5)
  arc A1 (2.3412, 7.1252) -> (-2.3412, 7.1252) centre (0, 0) ccw
  line L2 (15.6554, 7.884) -> (14.6554, 9.616)
  arc A2 (1, -17.5) -> (5, -13.5) centre (1, -13.5) ccw
  arc A3 (-5, -13.5) -> (-1, -17.5) centre (-1, -13.5) ccw
  arc A4 (-15.6554, 7.884) -> (-14.1913, 2.4199) centre (-12.1913, 5.884) ccw
  arc A5 (5, -5.5902) -> (7.3412, -1.535) centre (0, 0) ccw
  arc A6 (14.1913, 2.4199) -> (15.6554, 7.884) centre (12.1913, 5.884) ccw
  line L3 (-14.1913, 2.4199) -> (-7.3412, -1.535)
  arc A7 (-9.1913, 11.0801) -> (-14.6554, 9.616) centre (-11.1913, 7.616) ccw
  line L4 (-5, -5.5902) -> (-5, -13.5)
  line L5 (7.3412, -1.535) -> (14.1913, 2.4199)
  arc A8 (-7.3412, -1.535) -> (-5, -5.5902) centre (0, 0) ccw
  line L6 (-2.3412, 7.1252) -> (-9.1913, 11.0801)
  line L7 (5, -13.5) -> (5, -5.5902)
  line L8 (9.1913, 11.0801) -> (2.3412, 7.1252)
  circle A9 centre (0, 0) radius 65
  dimension "d1" = 130
  constraint concentric A1 A9
  measures "d1" diameter of A9
extrude "Extrude1" add sketch "Sketch1" against normal blind 6 makes body 1
sketch "Sketch2" plane through (0, 0, 0) normal (0, 0, 1) x (-1, 0, 0)
  line L0 (-2.3412, -7.1252) -> (-9.1913, -11.0801)
  arc A0 (-14.6554, -9.616) -> (-9.1913, -11.0801) centre (-11.1913, -7.616) ccw
  line L1 (-14.6554, -9.616) -> (-15.6554, -7.884)
  arc A1 (-14.1913, -2.4199) -> (-15.6554, -7.884) centre (-12.1913, -5.884) ccw
  line L2 (-14.1913, -2.4199) -> (-7.3412, 1.535)
  arc A2 (-5, 5.5902) -> (-7.3412, 1.535) centre (0, 0) ccw
  line L3 (-5, 5.5902) -> (-5, 13.5)
  arc A3 (-1, 17.5) -> (-5, 13.5) centre (-1, 13.5) ccw
  line L4 (-1, 17.5) -> (1, 17.5)
  arc A4 (5, 13.5) -> (1, 17.5) centre (1, 13.5) ccw
  line L5 (5, 13.5) -> (5, 5.5902)
  arc A5 (7.3412, 1.535) -> (5, 5.5902) centre (0, 0) ccw
  line L6 (7.3412, 1.535) -> (14.1913, -2.4199)
  arc A6 (15.6554, -7.884) -> (14.1913, -2.4199) centre (12.1913, -5.884) ccw
  line L7 (15.6554, -7.884) -> (14.6554, -9.616)
  arc A7 (9.1913, -11.0801) -> (14.6554, -9.616) centre (11.1913, -7.616) ccw
  line L8 (9.1913, -11.0801) -> (2.3412, -7.1252)
  arc A8 (-2.3412, -7.1252) -> (2.3412, -7.1252) centre (0, 0) ccw
  circle A9 centre (0, 0) radius 65
  circle A10 centre (0, 0) radius 27.5
  circle A11 centre (0, 0) radius 57.5
  dimension "d4" = 55
  dimension "d5" = 115
  constraint concentric A2 A10
  constraint concentric A2 A11
  measures "d4" diameter of A10
  measures "d5" diameter of A11
extrude "Extrude2" cut sketch "Sketch2" against normal blind 6 contours A11 bodies 1 makes body 2 at (62.0439, -6.0859, 0)
sketch "Sketch3" plane through (0, 0, 0) normal (0, 0, 1) x (-1, 0, 0)
  circle A0 centre (0, 0) radius 27.5
  line L0 (-2.3412, -7.1252) -> (-9.1913, -11.0801)
  arc A1 (-14.6554, -9.616) -> (-9.1913, -11.0801) centre (-11.1913, -7.616) ccw
  line L1 (-14.6554, -9.616) -> (-15.6554, -7.884)
  arc A2 (-14.1913, -2.4199) -> (-15.6554, -7.884) centre (-12.1913, -5.884) ccw
  line L2 (-14.1913, -2.4199) -> (-7.3412, 1.535)
  arc A3 (-5, 5.5902) -> (-7.3412, 1.535) centre (0, 0) ccw
  line L3 (-5, 5.5902) -> (-5, 13.5)
  arc A4 (-1, 17.5) -> (-5, 13.5) centre (-1, 13.5) ccw
  line L4 (-1, 17.5) -> (1, 17.5)
  arc A5 (5, 13.5) -> (1, 17.5) centre (1, 13.5) ccw
  line L5 (5, 13.5) -> (5, 5.5902)
  arc A6 (7.3412, 1.535) -> (5, 5.5902) centre (0, 0) ccw
  line L6 (7.3412, 1.535) -> (14.1913, -2.4199)
  arc A7 (15.6554, -7.884) -> (14.1913, -2.4199) centre (12.1913, -5.884) ccw
  line L7 (15.6554, -7.884) -> (14.6554, -9.616)
  arc A8 (9.1913, -11.0801) -> (14.6554, -9.616) centre (11.1913, -7.616) ccw
  line L8 (9.1913, -11.0801) -> (2.3412, -7.1252)
  arc A9 (-2.3412, -7.1252) -> (2.3412, -7.1252) centre (0, 0) ccw
  line L9 (0, -27.5) -> (0, -58) construction
  line L10 (0, -58) -> (-5, -58) construction
  line L11 (-5, -58) -> (-5, -26) construction
  line L12 (-5, -26) -> (5, -26) construction
  line L13 (5, -26) -> (5, -58) construction
  line L14 (0, -58) -> (5, -58) construction
  line L15 (5, -27.0416) -> (5, -58)
  line L16 (5, -58) -> (-5, -58)
  line L17 (-5, -58) -> (-5, -26)
  line L18 (-5, -26) -> (5, -26)
  line L19 (5, -27.0416) -> (5, -26)
  line L20 (25.0167, 8.6699) -> (20.0167, 17.3301)
  line L21 (20.9187, 17.8509) -> (20.0167, 17.3301)
  line L22 (20.9187, 17.8509) -> (47.7295, 33.3301)
  line L23 (52.7295, 24.6699) -> (25.0167, 8.6699) construction
  line L24 (47.7295, 33.3301) -> (52.7295, 24.6699)
  line L25 (-20.0167, 17.3301) -> (-25.0167, 8.6699)
  line L26 (-25.9187, 9.1907) -> (-25.0167, 8.6699)
  line L27 (-25.9187, 9.1907) -> (-52.7295, 24.6699)
  line L28 (-47.7295, 33.3301) -> (-20.0167, 17.3301) construction
  line L29 (-52.7295, 24.6699) -> (-47.7295, 33.3301)
  line L30 (-20.0167, 17.3301) -> (-47.7295, 33.3301)
  line L31 (25.0167, 8.6699) -> (52.7295, 24.6699)
  dimension "d9" = 360
  constraint coincident A0 L9.start
  constraint vertical L9
  constraint perpendicular L9 L10
  constraint perpendicular L10 L11
  constraint perpendicular L11 L12
  constraint perpendicular L12 L13
  constraint perpendicular L13 L14
  constraint coincident L13 L15.start
  constraint coincident A0 L15.start
  constraint perpendicular L11 L16
  constraint perpendicular L12 L19
extrude "Extrude3" add sketch "Sketch3" against normal blind 6 contours A0 L15 L16 L17 | A0 L22 L24 L31 | A0 L27 L29 L30 bodies 1 2
fillet "Fillet1" radius 4 12 edges at (-20.9187, -17.8509, -3) (-25.9187, -9.1907, -3) (-47.1078, -32.9712, -3) (-52.1078, -24.311, -3) (20.9187, -17.8509, -3) (25.9187, -9.1907, -3) (47.1078, -32.9712, -3) (52.1078, -24.311, -3) (5, 57.2822, -3) (-5, 57.2822, -3) (5, 27.0416, -3) (-5, 27.0416, -3) on bodies 1
sketch "Sketch4" plane through (0, 0, -6) normal (0, 0, -1) x (1, 0, 0)
  arc A0 (9.6729, -56.6806) -> (53.9232, 19.9633) centre (0, 0) ccw
  arc A1 (5, -52.7376) -> (9.6729, -56.6806) centre (9, -52.7376) ccw
  line L0 (5, -52.7376) -> (5, -30.1869)
  arc A2 (7.8571, -26.3537) -> (5, -30.1869) centre (9, -30.1869) ccw
  arc A3 (7.8571, -26.3537) -> (26.7515, 6.3723) centre (0, 0) ccw
  arc A4 (28.6426, 10.7633) -> (26.7515, 6.3723) centre (30.6426, 7.2992) ccw
  line L1 (28.6426, 10.7633) -> (48.1721, 22.0387)
  arc A5 (53.9232, 19.9633) -> (48.1721, 22.0387) centre (50.1721, 18.5746) ccw
  line L2 (43.1721, 30.6989) -> (23.6426, 19.4236)
  arc A6 (18.8944, 19.9813) -> (23.6426, 19.4236) centre (21.6426, 22.8877) ccw
  arc A7 (18.8944, 19.9813) -> (-18.8944, 19.9813) centre (0, 0) ccw
  arc A8 (-23.6426, 19.4236) -> (-18.8944, 19.9813) centre (-21.6426, 22.8877) ccw
  line L3 (-23.6426, 19.4236) -> (-43.1721, 30.6989)
  arc A9 (-44.2503, 36.7173) -> (-43.1721, 30.6989) centre (-41.1721, 34.163) ccw
  arc A10 (44.2503, 36.7173) -> (-44.2503, 36.7173) centre (0, 0) ccw
  arc A11 (43.1721, 30.6989) -> (44.2503, 36.7173) centre (41.1721, 34.163) ccw
  line L4 (-5, -30.1869) -> (-5, -52.7376)
  arc A12 (-9.6729, -56.6806) -> (-5, -52.7376) centre (-9, -52.7376) ccw
  arc A13 (-53.9232, 19.9633) -> (-9.6729, -56.6806) centre (0, 0) ccw
  arc A14 (-48.1721, 22.0387) -> (-53.9232, 19.9633) centre (-50.1721, 18.5746) ccw
  line L5 (-48.1721, 22.0387) -> (-28.6426, 10.7633)
  arc A15 (-26.7515, 6.3723) -> (-28.6426, 10.7633) centre (-30.6426, 7.2992) ccw
  arc A16 (-26.7515, 6.3723) -> (-7.8571, -26.3537) centre (0, 0) ccw
  arc A17 (-5, -30.1869) -> (-7.8571, -26.3537) centre (-9, -30.1869) ccw
  circle A18 centre (0, 0) radius 65
  line L6 (9.1913, -11.0801) -> (2.3412, -7.1252)
  arc A19 (-2.3412, -7.1252) -> (2.3412, -7.1252) centre (0, 0) ccw
  line L7 (-2.3412, -7.1252) -> (-9.1913, -11.0801)
  arc A20 (-14.6554, -9.616) -> (-9.1913, -11.0801) centre (-11.1913, -7.616) ccw
  line L8 (-14.6554, -9.616) -> (-15.6554, -7.884)
  arc A21 (-14.1913, -2.4199) -> (-15.6554, -7.884) centre (-12.1913, -5.884) ccw
  line L9 (-14.1913, -2.4199) -> (-7.3412, 1.535)
  arc A22 (-5, 5.5902) -> (-7.3412, 1.535) centre (0, 0) ccw
  line L10 (-5, 5.5902) -> (-5, 13.5)
  arc A23 (-1, 17.5) -> (-5, 13.5) centre (-1, 13.5) ccw
  line L11 (-1, 17.5) -> (1, 17.5)
  arc A24 (5, 13.5) -> (1, 17.5) centre (1, 13.5) ccw
  line L12 (5, 13.5) -> (5, 5.5902)
  arc A25 (7.3412, 1.535) -> (5, 5.5902) centre (0, 0) ccw
  line L13 (7.3412, 1.535) -> (14.1913, -2.4199)
  arc A26 (15.6554, -7.884) -> (14.1913, -2.4199) centre (12.1913, -5.884) ccw
  line L14 (15.6554, -7.884) -> (14.6554, -9.616)
  arc A27 (9.1913, -11.0801) -> (14.6554, -9.616) centre (11.1913, -7.616) ccw
  line L15 (2, -65.5) -> (-2, -65.5) construction
  line L16 (-2, -65.5) -> (-2, -64.5) construction
  line L17 (-2, -64.5) -> (2, -64.5) construction
  line L18 (2, -64.5) -> (2, -65.5) construction
  line L19 (2, -65.5) -> (-2, -64.5) construction
  line L20 (-2, -65.5) -> (2, -64.5) construction
  line L21 (-2, -64.5) -> (2, -64.5) construction
  line L22 (2, -64.5) -> (2, -65.5) construction
  line L23 (2, -65.5) -> (-2, -65.5) construction
  line L24 (-2, -65.5) -> (-2, -64.5) construction
  line L25 (-2, -64.5) -> (2, -64.5)
  line L26 (2, -64.5) -> (2, -65.5)
  line L27 (2, -65.5) -> (-2, -65.5)
  line L28 (-2, -65.5) -> (-2, -64.5)
  point P0 (0, -65)
  dimension "d14" = 1
  constraint horizontal L15
  constraint perpendicular L15 L16
  constraint parallel L15 L17
  constraint parallel L16 L18
  constraint coincident L19 P0
  constraint coincident L20 P0
  constraint coincident A18 P0
  constraint horizontal L21
  constraint vertical L22
  constraint horizontal L23
  constraint vertical L24
  constraint horizontal L25
  constraint vertical L26
  constraint horizontal L27
  constraint vertical L28
  measures "d14" distance of L15.end L16.end
extrude "Extrude4" cut sketch "Sketch4" against normal blind 6 contours A18 L25 L26 L28 picked at (-0.2223, -64.6655) bodies 1
pattern_circular "C-Pattern1" count 42 over 360 about axis through (0, 0, 1.75) along (0, 0, 1) of "Extrude4"